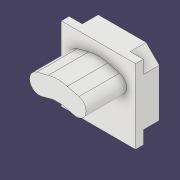
# Autodesk Inventor part: Base
Saved by Autodesk Inventor 2017 SP1 (Build 210196100, 196)
## iProperties
Created: 2018-03-03
Part Number: Base
Material: ABS Plastic
Document SubType Name: Modeling
Designer: Zach
Density: 1.06 g/cm^3
Appearance: CR White
Author: Zach
Autodesk Inventor part; units mm, degrees
ref_plane "YZ Plane" through (0, 0, 0) normal (1, 0, 0) x (0, 1, 0)
ref_plane "XZ Plane" through (0, 0, 0) normal (0, 1, 0) x (-1, 0, 0)
ref_plane "XY Plane" through (0, 0, 0) normal (0, 0, 1) x (1, 0, 0)
sketch "Sketch1" plane through (0, 0, 0) normal (0, 0, 1) x (1, 0, 0)
  line L0 (-310, 185.5) -> (310, 185.5)
  line L1 (310, 185.5) -> (310, -434.5)
  line L2 (310, -434.5) -> (-310, -434.5)
  line L3 (-310, -434.5) -> (-310, 185.5)
  point P0 (0, 0)
  point P1 (0, 185.5)
  dimension "d0" = 620
  dimension "d1" = 620
  dimension "d2" = 185.5
  constraints: 8 end point, 2 parallel, 1 horizontal, 1 midpoint, 1 perpendicular, 1 vertical alignment
  measures "d0" distance of L1.end L2.end
  measures "d1" distance of L0.end L1.end
  measures "d2" distance from line of L0 point (0, 0)
extrude "Extrusion1" add sketch "Sketch1" along normal mid plane 198
sketch "Sketch2" plane through (0, 0, -99) normal (0, 0, -1) x (-1, 0, 0)
  line L0 (-310, 185.5) -> (310, 185.5) projected
  line L1 (-310, 185.5) -> (-310, 75.5)
  line L2 (-310, -434.5) -> (-310, 185.5) projected
  line L3 (-310, 75.5) -> (-200, 185.5)
  line L4 (-310, 185.5) -> (-200, 185.5)
  line L5 (-310, -124.5) -> (0, -124.5)
  line L6 (0, -124.5) -> (0, 185.5)
  line L7 (-310, -434.5) -> (-310, -324.5)
  line L8 (-310, -434.5) -> (-200, -434.5)
  line L9 (-200, -434.5) -> (-310, -324.5)
  line L10 (310, -434.5) -> (200, -434.5)
  line L11 (310, -434.5) -> (310, -324.5)
  line L12 (310, -324.5) -> (200, -434.5)
  line L13 (310, 185.5) -> (310, 75.5)
  line L14 (310, 185.5) -> (200, 185.5)
  line L15 (200, 185.5) -> (310, 75.5)
  point P0 (0, 0)
  dimension "d5" = 110
  dimension "d6" = 110
  dimension "d9" = 360
  constraints: 28 end point, 2 midpoint, 1 collinear, 1 horizontal, 1 point on line, 1 vertical, 25 other
  measures "d5" distance of L0.start L1.end
  measures "d6" distance of L0.start L3.end
extrude "Extrusion2" cut sketch "Sketch2" against normal blind 133 contours L0 L13 L15 | L9 L8 L2 | L0 L3 L1 | L10 L12 L11
sketch "Sketch3" plane through (0, 0, 99) normal (0, 0, 1) x (1, 0, 0)
  circle A0 centre (-155.8871, -26.656) radius 80 construction
  line L0 (-176.5926, 50.6181) -> (-80, 76.5)
  line L1 (-135.1815, -103.93) -> (-38.589, -78.0481)
  line L2 (-80, 76.5) -> (-38.589, -78.0481) construction
  line L3 (-80, 76.5) -> (80, 76.5) construction
  line L4 (80, 76.5) -> (38.589, -78.0481) construction
  line L5 (-38.589, -78.0481) -> (38.589, -78.0481)
  circle A1 centre (155.8871, -26.656) radius 80 construction
  line L6 (38.589, -78.0481) -> (135.1815, -103.93)
  line L7 (80, 76.5) -> (176.5926, 50.6181)
  arc A2 (-176.5926, 50.6181) -> (-135.1815, -103.93) centre (-155.8871, -26.656) ccw
  arc A3 (135.1815, -103.93) -> (176.5926, 50.6181) centre (155.8871, -26.656) ccw
  circle A4 centre (-155.8871, -26.656) radius 5.25
  circle A5 centre (155.8871, -26.656) radius 5.25
  line L8 (-106.5, 56.5) -> (-106.5, -56.5)
  line L9 (-106.5, -56.5) -> (106.5, -56.5)
  line L10 (106.5, -56.5) -> (106.5, 56.5)
  line L11 (106.5, 56.5) -> (-106.5, 56.5)
  arc A6 (80, 76.5) -> (-80, 76.5) centre (0, -228.172) ccw
  circle A7 centre (0, 71.664) radius 5.25
  line L12 (310, -434.5) -> (310, 185.5) construction
  line L13 (310, 185.5) -> (-310, 185.5) construction
  line L14 (0, 185.5) -> (0, 0) construction
  line L15 (0, 0) -> (310, 0) construction
  line L16 (310, 75.5) -> (310, -324.5) construction
  line L17 (0, -78.0481) -> (0, -56.5)
  point P0 (0, 76.5)
  point P1 (-106.5, 0)
  dimension "d32" = 160
  dimension "d33" = 100
  dimension "d34" = 100
  dimension "d35" = 160
  dimension "d36" = 160
  dimension "d37" = 160
  dimension "d38" = 75
  dimension "d39" = 75
  dimension "d40" = 160
  dimension "d41" = 100
  dimension "d42" = 100
  dimension "d43" = 10.5
  dimension "d44" = 10.5
  dimension "d45" = 113
  dimension "d46" = 213
  dimension "d47" = 20
  dimension "d48" = 315
  dimension "d49" = 10.5
  dimension "d50" = 15.164
  dimension "d51" = 185.5
  constraints: 30 end point, 10 point on circle, 8 centre point, 8 tangent, 5 midpoint, 4 coincident, 3 perpendicular, 2 parallel, 2 point on line, 2 vertical alignment, 1 horizontal alignment, 1 vertical
  measures "d32" diameter of A0
  measures "d33" distance of L0.end L0.start
  measures "d34" distance of L5.start L1.start
  measures "d35" distance of L0.end L5.start
  measures "d36" distance of L0.end L7.start
  measures "d37" distance of L7.start L6.start
  measures "d38" angle of L3 L2
  measures "d39" angle of L3 L4
  measures "d40" diameter of A1
  measures "d41" distance of L6.start L6.end
  measures "d42" distance of L7.start L7.end
  measures "d43" diameter of A4
  measures "d44" diameter of A5
  measures "d45" distance of L10.end L10.start
  measures "d46" distance of L10.start L8.end
  measures "d47" distance between parallel lines of L3 L11
  measures "d48" radius of A6
  measures "d49" diameter of A7
  measures "d50" distance from line of L11 A7.centre
  measures "d51" distance of L14.start L14.end
extrude "Extrusion3" add sketch "Sketch3" along normal blind 339 contours L9 L8 L11 L10 | L0 A6 L7 A3 L6 L5 L1 A2 | A4 | A5 | A7
body "Solid1"
